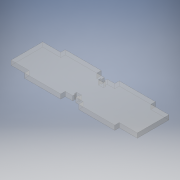
# Autodesk Inventor part: Interrupter_Side
Saved by Autodesk Inventor 2016 (Build 200138000, 138)
## iProperties
Created: 2018-05-24
Part Number: Interrupter_Side
Material: Polycarbonate, Clear
Document SubType Name: Modeling
Designer: Phil Erle
Density: 1.2 g/cm^3
Appearance: Polycarbonate - Clear
Author: Phil Erle
Autodesk Inventor part; units mm, degrees
ref_plane "YZ Plane" through (0, 0, 0) normal (1, 0, 0) x (0, 1, 0)
ref_plane "XZ Plane" through (0, 0, 0) normal (0, 1, 0) x (-1, 0, 0)
ref_plane "XY Plane" through (0, 0, 0) normal (0, 0, 1) x (1, 0, 0)
sketch "Sketch2" plane through (0, 0, 0) normal (0, 0, 1) x (1, 0, 0)
  line L0 (-70, 17.5) -> (-70, -17.5)
  line L1 (-70, -17.5) -> (-50, -17.5)
  line L2 (-50, -17.5) -> (-50, -22.5)
  line L3 (-50, -22.5) -> (-10, -22.5)
  line L4 (-10, -22.5) -> (-10, -17.5)
  line L5 (-10, -17.5) -> (10, -17.5)
  line L6 (10, -17.5) -> (10, -22.5)
  line L7 (10, -22.5) -> (50, -22.5)
  line L8 (50, -22.5) -> (50, -17.5)
  line L9 (50, -17.5) -> (70, -17.5)
  line L10 (70, -17.5) -> (70, 17.5)
  line L11 (70, 17.5) -> (50, 17.5)
  line L12 (50, 17.5) -> (50, 22.5)
  line L13 (50, 22.5) -> (10, 22.5)
  line L14 (10, 22.5) -> (10, 17.5)
  line L15 (10, 17.5) -> (-10, 17.5)
  line L16 (-10, 17.5) -> (-10, 22.5)
  line L17 (-10, 22.5) -> (-50, 22.5)
  line L18 (-50, 22.5) -> (-50, 17.5)
  line L19 (-50, 17.5) -> (-70, 17.5)
  point P0 (0, 0)
  point P1 (0, 17.5)
  point P2 (0, -17.5)
  point P3 (-70, 0)
  point P4 (70, 0)
  dimension "d11" = 5
  dimension "d12" = 35
  dimension "d13" = 20
  dimension "d14" = 40
  dimension "d15" = 140
  dimension "d16" = 40
  dimension "d17" = 5
  dimension "d18" = 70
  constraints: 40 end point, 15 point on line, 12 perpendicular, 4 midpoint, 3 horizontal alignment, 2 vertical alignment, 1 vertical
  measures "d11" distance of L11.end L12.end
  measures "d12" distance of L9.end L10.end
  measures "d13" distance between parallel lines of L16 L14
  measures "d14" distance of L12.end L13.end
  measures "d15" distance between parallel lines of L10 L0
  measures "d16" distance of L16.end L17.end
  measures "d17" distance of L1.end L2.end
  measures "d18" distance from line of point (0, 0) L0
extrude "Extrusion1" add sketch "Sketch2" along normal blind 5
sketch "Sketch3" plane through (0, 0, 5) normal (0, 0, 1) x (1, 0, 0)
  line L0 (10, 17.5) -> (-10, 17.5) projected
  line L1 (-10, -17.5) -> (10, -17.5) projected
  line L2 (1.6, 17.5) -> (-1.6, 17.5)
  line L3 (-1.6, 17.5) -> (-1.6, 14.4)
  line L4 (-1.6, 14.4) -> (-2.75, 14.4)
  line L5 (-2.75, 14.4) -> (-2.75, 12)
  line L6 (-2.75, 12) -> (2.75, 12)
  line L7 (2.75, 12) -> (2.75, 14.4)
  line L8 (2.75, 14.4) -> (1.6, 14.4)
  line L9 (1.6, 17.5) -> (1.6, 14.4)
  line L10 (-1.6, -17.5) -> (1.6, -17.5)
  line L11 (1.6, -17.5) -> (1.6, -14.4)
  line L12 (1.6, -14.4) -> (2.75, -14.4)
  line L13 (2.75, -14.4) -> (2.75, -12)
  line L14 (2.75, -12) -> (-2.75, -12)
  line L15 (-2.75, -12) -> (-2.75, -14.4)
  line L16 (-2.75, -14.4) -> (-1.6, -14.4)
  line L17 (-1.6, -14.4) -> (-1.6, -17.5)
  point P0 (0, 0)
  point P1 (0, 17.5)
  point P2 (0, 12)
  point P3 (0, -17.5)
  point P4 (0, -12)
  point P5 (0, 17.5)
  dimension "d21" = 3.2
  dimension "d22" = 2.4
  dimension "d23" = 2.4
  dimension "d24" = 3.2
  dimension "d25" = 5.5
  dimension "d26" = 5.5
  dimension "d27" = 5.5
  dimension "d28" = 5.5
  constraints: 32 end point, 10 perpendicular, 8 point on line, 5 midpoint, 5 vertical alignment, 2 vertical
  measures "d21" distance between parallel lines of L17 L11
  measures "d22" distance of L12.end L13.end
  measures "d23" distance of L6.end L7.end
  measures "d24" distance between parallel lines of L3 L9
  measures "d25" distance of L5.end L6.end
  measures "d26" distance of L13.end L14.end
  measures "d27" distance between parallel lines of L0 L6
  measures "d28" distance between parallel lines of L1 L14
extrude "Extrusion2" cut sketch "Sketch3" against normal blind 5
equation "\"d18\" = 0.5 * d15"
body "Solid1"
